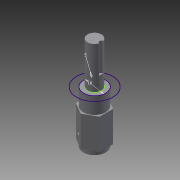
# Autodesk Inventor part: AnyaKicsi
Saved by Autodesk Inventor 2015 (Build 190159000, 159)
## iProperties
Created: 2014-08-26
Part Number: AnyaKicsi
Material: Generic
Document SubType Name: Modeling
Designer: laca
Density: 1 g/cm^3
Appearance: Default
Mass: 8.24855 g
Surface Area: 45.6248 cm^2
Volume: 8.24855 cm^3
Author: laca
Autodesk Inventor part; units mm, degrees
ref_plane "YZ Plane" through (0, 0, 0) normal (1, 0, 0) x (0, 1, 0)
ref_plane "XZ Plane" through (0, 0, 0) normal (0, 1, 0) x (-1, 0, 0)
ref_plane "XY Plane" through (0, 0, 0) normal (0, 0, 1) x (1, 0, 0)
sketch "Sketch1" plane through (0, 0, 0) normal (0, 1, 0) x (-1, 0, 0)
  line L0 (8.5475, 4.8243) -> (8.4517, -4.9902)
  line L1 (8.4517, -4.9902) -> (-0.0957, -9.8145)
  line L2 (-0.0957, -9.8145) -> (-8.5475, -4.8243)
  line L3 (-8.5475, -4.8243) -> (-8.4517, 4.9902)
  line L4 (-8.4517, 4.9902) -> (0.0957, 9.8145)
  line L5 (0.0957, 9.8145) -> (8.5475, 4.8243)
  circle A0 centre (0, 0) radius 5
  dimension "d0" = 17
  dimension "d1" = 10
  constraints: 12 end point, 2 coincident, 1 centre point, 13 other
  measures "d0" distance between parallel lines of L2 L5
  measures "d1" diameter of A0
extrude "Extrusion1" add sketch "Sketch1" along normal blind 37
sketch "Sketch2" plane through (0, 37, 0) normal (0, 1, 0) x (1, 0, 0)
  circle A0 centre (0, 0) radius 8
  circle A1 centre (0, 0) radius 13
  circle A2 centre (0, 0) radius 5
  dimension "d4" = 16
  dimension "d5" = 5
  constraints: 3 centre point, 3 coincident
  measures "d4" diameter of A0
  measures "d5" radial gap between concentric circles of A1 A0
extrude "Extrusion2" cut sketch "Sketch2" against normal blind 12 contours A1
sketch "Sketch3" plane through (0, 0, 0) normal (0, -1, 0) x (1, 0, 0)
  circle A0 centre (0, 0) radius 8
  circle A1 centre (0, 0) radius 13
  dimension "d9" = 16
  dimension "d10" = 5
  constraints: 2 centre point, 2 coincident
  measures "d9" diameter of A0
  measures "d10" radial gap between concentric circles of A1 A0
extrude "Extrusion3" cut sketch "Sketch3" against normal blind 3
sketch "Sketch9" plane through (0.0957, 3, -9.8145) normal (0.5084, 0, -0.8611) x (-0.8611, 0, -0.5084)
  circle A0 centre (-4.9075, 7) radius 1.5
  line L0 (-9.815, 0) -> (-9.815, 22) projected
  line L1 (0, 0) -> (0, 22) projected
  point P0 (-4.9075, -3)
  dimension "d31" = 3
  dimension "d32" = 9.8149
  dimension "d33" = 4.9075
  dimension "d34" = 10
  constraints: 1 centre point
  measures "d31" diameter of A0
  measures "d32" distance between parallel lines of L0 L1
  measures "d33" distance from line of L1 A0.centre
  measures "d34" distance of point (-4.907, -3) A0.centre
extrude "Extrusion5" cut sketch "Sketch9" against normal through all
extrude "Extrusion6" add sketch "Sketch2" along normal blind 30 and the other way blind 5 contours A2
sketch "Sketch10" plane through (0, 67, 0) normal (0, 1, 0) x (1, 0, 0)
  circle A0 centre (0, 0) radius 5 projected
  circle A1 centre (5, 0) radius 1.5
  dimension "d45" = 3
  constraints: 1 centre point, 1 horizontal alignment, 1 other
  measures "d45" diameter of A1
extrude "Extrusion7" cut sketch "Sketch10" against normal blind 20 contours A0 A1 | A0 A1 picked at (4.5056, -0.2843) picked at (5.4323, -0.4031)
equation "\"d33\" = 0.5 * d32"
body "Solid1"
